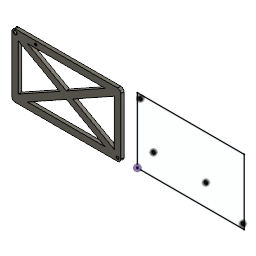
psu_mount_on_baseplate v1 (Autodesk Fusion 360 design; units mm, degrees)
Autodesk Fusion 360 part; units mm, degrees
sketch "Sketch1" plane through (0, 0, 0) normal (0, 0, 1) x (1, 0, 0)
  line L0 (100, 125) -> (-100, 125)
  line L1 (-100, 125) -> (-100, -125)
  line L2 (-100, -125) -> (100, -125)
  line L3 (100, -125) -> (100, 125)
  line L4 (100, 125) -> (-100, -125) construction
  line L5 (-100, 125) -> (100, -125) construction
  line L6 (-100, 125) -> (100, 125)
  line L7 (100, 125) -> (100, 129)
  line L8 (100, 129) -> (-100, 129)
  line L9 (-100, 129) -> (-100, 125)
  line L10 (-100, -125) -> (100, -125)
  line L11 (100, -125) -> (100, -129)
  line L12 (100, -129) -> (-100, -129)
  line L13 (-100, -129) -> (-100, -125)
  line L14 (100, 125) -> (104, 125)
  line L15 (104, 125) -> (104, -125)
  line L16 (104, -125) -> (100, -125)
  line L17 (100, -125) -> (100, 125)
  line L18 (-100, 125) -> (-104, 125)
  line L19 (-104, 125) -> (-104, -125)
  line L20 (-104, -125) -> (-100, -125)
  line L21 (-100, -125) -> (-100, 125)
  line L22 (-80, -53.8) -> (-80, 2.2) construction
  circle A0 centre (-80, -53.8) radius 1.65 construction
  circle A1 centre (-80, 2.2) radius 1.65 construction
  line L23 (-61.0622, -1) -> (-98.9378, -1) construction
  line L24 (-98.9378, -1) -> (-98.9378, -50.6) construction
  line L25 (-98.9378, -50.6) -> (-61.0622, -50.6) construction
  line L26 (-61.0622, -50.6) -> (-61.0622, -1) construction
  line L27 (-61.0622, -1) -> (-98.9378, -50.6) construction
  line L28 (-98.9378, -1) -> (-61.0622, -50.6) construction
  line L29 (-30.5, 49.5) -> (98.5, 49.5) construction
  line L30 (98.5, 49.5) -> (98.5, -47.5) construction
  line L31 (98.5, -47.5) -> (-30.5, -47.5) construction
  line L32 (-30.5, -47.5) -> (-30.5, 49.5) construction
  circle A2 centre (-28, 43) radius 1.65
  circle A3 centre (94, -42) radius 1.65
  line L33 (-100, 125) -> (-85.5, 125)
  line L34 (-85.5, 125) -> (-85.5, 116)
  line L35 (-85.5, 116) -> (-100, 116)
  line L36 (-100, 116) -> (-100, 125)
  line L37 (100, 125) -> (85.5, 125)
  line L38 (85.5, 125) -> (85.5, 116)
  line L39 (85.5, 116) -> (100, 116)
  line L40 (100, 116) -> (100, 125)
  line L41 (-100, -125) -> (-85.5, -125)
  line L42 (-85.5, -125) -> (-85.5, -116)
  line L43 (-85.5, -116) -> (-100, -116)
  line L44 (-100, -116) -> (-100, -125)
  line L45 (100, -125) -> (85.5, -125)
  line L46 (85.5, -125) -> (85.5, -116)
  line L47 (85.5, -116) -> (100, -116)
  line L48 (100, -116) -> (100, -125)
  line L49 (-100, 100) -> (-104, 100)
  line L50 (100, 100) -> (104, 100)
  line L51 (-100, -100) -> (-104, -100)
  line L52 (100, -100) -> (104, -100)
  line L53 (-85.5, 125) -> (-85.5, 129)
  line L54 (85.5, 125) -> (85.5, 129)
  line L55 (-85.5, -125) -> (-85.5, -129)
  line L56 (85.5, -125) -> (85.5, -129)
  line L57 (-115, -140) -> (-75, -140) construction
  line L58 (-75, -140) -> (-75, -87) construction
  line L59 (-75, -87) -> (-115, -87) construction
  line L60 (-115, -87) -> (-115, -140) construction
  line L61 (-63.3606, -140) -> (-21.3606, -140) construction
  line L62 (-21.3606, -140) -> (-21.3606, -53.8) construction
  line L63 (-21.3606, -53.8) -> (-63.3606, -53.8) construction
  line L64 (-63.3606, -53.8) -> (-63.3606, -140) construction
  line L65 (-100, 0) -> (-118.2487, 0) construction
  circle A4 centre (0, 0) radius 152.5
  circle A5 centre (-85, -72) radius 1.65
  line L66 (-85, -72) -> (85, -72) construction
  line L67 (85, -72) -> (85, 72) construction
  line L68 (85, 72) -> (-85, 72) construction
  line L69 (-85, 72) -> (-85, -72) construction
  circle A6 centre (85, 72) radius 1.65
  circle A7 centre (85, -72) radius 1.65
  circle A8 centre (-85, 72) radius 1.65
  point P0 (-80, -25.8)
  dimension "d1" = 200
  dimension "d2" = 250
  dimension "d3" = 4
  dimension "d4" = 4
  dimension "d5" = 4
  dimension "d6" = 4
  dimension "d7" = 20
  dimension "d8" = 56
  dimension "d10" = 3.3
  dimension "d11" = 37.8755
  dimension "d12" = 49.6
  dimension "d13" = 2.5
  dimension "d14" = 6.5
  dimension "d15" = 3.3
  dimension "d16" = 5.5
  dimension "d17" = 4.5
  dimension "d18" = 129
  dimension "d19" = 97
  dimension "d20" = 1.5
  dimension "d21" = 14.5
  dimension "d22" = 9
  dimension "d23" = 14.5
  dimension "d24" = 9
  dimension "d25" = 14.5
  dimension "d26" = 14.5
  dimension "d27" = 9
  dimension "d28" = 9
  dimension "d29" = 25
  dimension "d30" = 25
  dimension "d31" = 25
  dimension "d32" = 25
  dimension "d33" = 40
  dimension "d34" = 53
  dimension "d35" = 15
  dimension "d36" = 15
  dimension "d37" = 3.3
  dimension "d38" = 86.2
  dimension "d39" = 42
  dimension "d40" = 1
  dimension "d50" = 305
  dimension "d51" = 3.3
  dimension "d52" = 15
  dimension "d53" = 15
  dimension "d54" = 15
  dimension "d55" = 53
  dimension "d56" = 53
  dimension "d57" = 170
  dimension "d58" = 144
  dimension "d60" = 47.5
  dimension "d61" = 49.5
  constraint horizontal L0
  constraint perpendicular L0 L1
  constraint parallel L0 L2
  constraint parallel L1 L3
  constraint coincident L4 A4.centre
  constraint coincident L5 A4.centre
  constraint coincident A4.centre origin
  constraint horizontal L6
  constraint vertical L7
  constraint horizontal L8
  constraint vertical L9
  constraint horizontal L10
  constraint vertical L11
  constraint horizontal L12
  constraint vertical L13
  constraint horizontal L14
  constraint vertical L15
  constraint horizontal L16
  constraint vertical L17
  constraint horizontal L18
  constraint vertical L19
  constraint horizontal L20
  constraint vertical L21
  constraint coincident L22.start A0.centre
  constraint coincident L22.end A1.centre
  constraint equal A0 A1
  constraint horizontal L23
  constraint perpendicular L23 L24
  constraint parallel L23 L25
  constraint parallel L24 L26
  constraint coincident L27 P0
  constraint coincident L28 P0
  constraint midpoint L22 P0
  constraint collinear L2 L20
  constraint collinear L11 L17
  constraint collinear L7 L17
  constraint horizontal L29
  constraint vertical L30
  constraint horizontal L31
  constraint vertical L32
  constraint equal A2 A3
  constraint horizontal L33
  constraint vertical L34
  constraint horizontal L35
  constraint vertical L36
  constraint horizontal L37
  constraint vertical L38
  constraint horizontal L39
  constraint vertical L40
  constraint horizontal L41
  constraint vertical L42
  constraint horizontal L43
  constraint vertical L44
  constraint horizontal L45
  constraint vertical L46
  constraint horizontal L47
  constraint vertical L48
  constraint coincident L1 L49.start
  constraint coincident L19 L49.end
  constraint perpendicular L19 L49
  constraint coincident L3 L50.start
  constraint coincident L15 L50.end
  constraint perpendicular L15 L50
  constraint coincident L21 L51.start
  constraint coincident L19 L51.end
  constraint perpendicular L19 L51
  constraint coincident L17 L52.start
  constraint coincident L15 L52.end
  constraint perpendicular L15 L52
  constraint coincident L8 L53.end
  constraint perpendicular L8 L53
  constraint coincident L8 L54.end
  constraint perpendicular L8 L54
  constraint coincident L12 L55.end
  constraint perpendicular L12 L55
  constraint coincident L12 L56.end
  constraint perpendicular L12 L56
  constraint horizontal L57
  constraint vertical L58
  constraint horizontal L59
  constraint vertical L60
  constraint horizontal L61
  constraint vertical L62
  constraint horizontal L63
  constraint vertical L64
  constraint vertical L22
  constraint midpoint L21 L65.start
  constraint perpendicular L19 L65
  constraint collinear L57 L61
  constraint horizontal L66
  constraint vertical L67
  constraint horizontal L68
  constraint vertical L69
  constraint coincident A5.centre L66.start
  constraint coincident L67.end L68.start
  constraint coincident L66.end L67.start
  constraint coincident L68.end L69.start
  constraint equal A6 A8
  constraint equal A5 A7
  constraint equal A6 A7
  measures "d1" distance of L0.start L0.end
  measures "d2" distance of L0.start L2.end
  measures "d3" distance of L0 L8
  measures "d4" distance of L2.end L11.end
  measures "d5" distance of L0.start L14.end
  measures "d6" distance of L0.end L18.end
  measures "d7" distance of L1 L22.start
  measures "d8" distance of L22.start L22.end
  measures "d10" diameter of A1
  measures "d11" distance of L23.start L23.end
  measures "d12" distance of L23.start L25.end
  measures "d13" distance of L32 A2.centre
  measures "d14" distance of L29 A2.centre
  measures "d15" diameter of A2
  measures "d16" distance of L31 A3.centre
  measures "d17" distance of L30 A3.centre
  measures "d18" distance of L29.start L29.end
  measures "d19" distance of L29.end L30.end
  measures "d20" distance of L17 L30
  measures "d21" distance of L34.end L35.end
  measures "d22" distance of L33.end L34.end
  measures "d23" distance of L38.end L39.end
  measures "d24" distance of L37.end L38.end
  measures "d25" distance of L42.end L43.end
  measures "d26" distance of L46.end L47.end
  measures "d27" distance of L41.end L42.end
  measures "d28" distance of L45.end L46.end
  measures "d29" distance of L20 L51
  measures "d30" distance of L18 L49
  measures "d31" distance of L14 L50
  measures "d32" distance of L10 L52
  measures "d33" distance of L57.start L57.end
  measures "d34" distance of L57.start L59.end
  measures "d35" distance of L10 L57
  measures "d36" distance of L21 L60
  measures "d37" diameter of A3
  measures "d38" distance of L61.end L62.end
  measures "d39" distance of L61.start L61.end
  measures "d40" distance of L23 L65
  measures "d50" diameter of A4
  measures "d51" diameter of A5
  measures "d52" distance of L1 A5.centre
  measures "d53" distance of L59 A5.centre
  measures "d54" distance of L17 L67
  measures "d55" distance of L10 L66
  measures "d56" distance of L6 L68
  measures "d57" distance of L67.end L68.end
  measures "d58" distance of L66.end L67.end
  measures "d60" distance of L31 L65
  measures "d61" distance of L29 L65
extrude "Extrude1" add sketch "Sketch1" along normal blind 3 contours L0 L1 L2 L3 L6 L10 L17 L21 L34 L35 L38 L39 L42 L43 L46 L47 A4 | L0 L6 L8 L53 L54 A4 | L3 L15 L17 L50 L52 | L1 L19 L21 L49 L51 | L2 L10 L12 L55 L56 A4 makes body 1
sketch "Sketch2" plane through (0, 0, 3) normal (0, 0, 1) x (1, 0, 0)
  circle A0 centre (85, -72) radius 1.65
  circle A1 centre (-85, -72) radius 1.65
  circle A2 centre (85, 72) radius 1.65
  circle A3 centre (94, -42) radius 1.65
  circle A4 centre (-85, 72) radius 1.65
  circle A5 centre (-28, 43) radius 1.65
  line L0 (100, 100) -> (100, 115.1358)
  arc A6 (100, 115.1358) -> (98.9962, 116) centre (0, 0) ccw
  line L1 (98.9962, 116) -> (85.5, 116)
  line L2 (85.5, 116) -> (85.5, 126.2775)
  arc A7 (85.5, 126.2775) -> (81.3342, 129) centre (0, 0) ccw
  line L3 (81.3342, 129) -> (-81.3342, 129)
  arc A8 (-81.3342, 129) -> (-85.5, 126.2775) centre (0, 0) ccw
  line L4 (-85.5, 126.2775) -> (-85.5, 116)
  line L5 (-85.5, 116) -> (-98.9962, 116)
  arc A9 (-98.9962, 116) -> (-100, 115.1358) centre (0, 0) ccw
  line L6 (-100, 115.1358) -> (-100, 100)
  line L7 (-100, 100) -> (-104, 100)
  line L8 (-104, 100) -> (-104, -100)
  line L9 (-104, -100) -> (-100, -100)
  line L10 (-100, -100) -> (-100, -115.1358)
  arc A10 (-100, -115.1358) -> (-98.9962, -116) centre (0, 0) ccw
  line L11 (-98.9962, -116) -> (-85.5, -116)
  line L12 (-85.5, -116) -> (-85.5, -126.2775)
  arc A11 (-85.5, -126.2775) -> (-81.3342, -129) centre (0, 0) ccw
  line L13 (-81.3342, -129) -> (81.3342, -129)
  arc A12 (81.3342, -129) -> (85.5, -126.2775) centre (0, 0) ccw
  line L14 (85.5, -126.2775) -> (85.5, -116)
  line L15 (85.5, -116) -> (98.9962, -116)
  arc A13 (98.9962, -116) -> (100, -115.1358) centre (0, 0) ccw
  line L16 (100, -115.1358) -> (100, -100)
  line L17 (100, -100) -> (104, -100)
  line L18 (104, -100) -> (104, 100)
  line L19 (104, 100) -> (100, 100)
  line L20 (-10, 129) -> (10, 129)
  line L21 (10, 129) -> (10, 111)
  line L22 (8, 109) -> (-8, 109)
  line L23 (-10, 111) -> (-10, 129)
  arc A14 (-10, 111) -> (-8, 109) centre (-8, 111) ccw
  arc A15 (8, 109) -> (10, 111) centre (8, 111) ccw
  point P0 (10, 109)
  point P1 (-10, 109)
  dimension "d62" = 20
  dimension "d63" = 20
  dimension "d64" = 2
  constraint horizontal L20
  constraint vertical L21
  constraint horizontal L22
  constraint vertical L23
  constraint coincident L3 L20.start
  constraint midpoint L3 L20
  constraint coincident P1 L22
  constraint coincident P1 L23
  constraint tangent L22 A14
  constraint tangent L23 A14
  constraint coincident P0 L21
  constraint coincident P0 L22
  constraint tangent L21 A15
  constraint tangent L22 A15
  constraint equal A14 A15
  measures "d62" distance of L20.start P1
  measures "d63" distance of P0 P1
  measures "d64" radius of A14
extrude "Extrude2" cut sketch "Sketch2" against normal blind 3 contours L3 L20 L21 L22 L23 A14 A15 bodies 1
fillet "Fillet4" radius 2 2 edges at (-10, 129, 1.5) (10, 129, 1.5) on bodies 1
sketch "Sketch3" plane through (0, 0, 3) normal (0, 0, 1) x (1, 0, 0)
  arc A0 (12, 129) -> (10, 127) centre (12, 127) ccw
  line L0 (10, 127) -> (10, 111)
  arc A1 (8, 109) -> (10, 111) centre (8, 111) ccw
  line L1 (8, 109) -> (-8, 109)
  arc A2 (-10, 111) -> (-8, 109) centre (-8, 111) ccw
  line L2 (-10, 111) -> (-10, 127)
  arc A3 (-10, 127) -> (-12, 129) centre (-12, 127) ccw
  line L3 (-12, 129) -> (-81.3342, 129)
  arc A4 (-81.3342, 129) -> (-85.5, 126.2775) centre (0, 0) ccw
  line L4 (-85.5, 126.2775) -> (-85.5, 116)
  line L5 (-85.5, 116) -> (-98.9962, 116)
  arc A5 (-98.9962, 116) -> (-100, 115.1358) centre (0, 0) ccw
  line L6 (-100, 115.1358) -> (-100, 100)
  line L7 (-100, 100) -> (-104, 100)
  line L8 (-104, 100) -> (-104, -100)
  line L9 (-104, -100) -> (-100, -100)
  line L10 (-100, -100) -> (-100, -115.1358)
  arc A6 (-100, -115.1358) -> (-98.9962, -116) centre (0, 0) ccw
  line L11 (-98.9962, -116) -> (-85.5, -116)
  line L12 (-85.5, -116) -> (-85.5, -126.2775)
  arc A7 (-85.5, -126.2775) -> (-81.3342, -129) centre (0, 0) ccw
  line L13 (-81.3342, -129) -> (81.3342, -129)
  arc A8 (81.3342, -129) -> (85.5, -126.2775) centre (0, 0) ccw
  line L14 (85.5, -126.2775) -> (85.5, -116)
  line L15 (85.5, -116) -> (98.9962, -116)
  arc A9 (98.9962, -116) -> (100, -115.1358) centre (0, 0) ccw
  line L16 (100, -115.1358) -> (100, -100)
  line L17 (100, -100) -> (104, -100)
  line L18 (104, -100) -> (104, 100)
  line L19 (104, 100) -> (100, 100)
  line L20 (100, 100) -> (100, 115.1358)
  arc A10 (100, 115.1358) -> (98.9962, 116) centre (0, 0) ccw
  line L21 (98.9962, 116) -> (85.5, 116)
  line L22 (85.5, 116) -> (85.5, 126.2775)
  arc A11 (85.5, 126.2775) -> (81.3342, 129) centre (0, 0) ccw
  line L23 (81.3342, 129) -> (12, 129)
  circle A12 centre (85, -72) radius 1.65
  circle A13 centre (-85, -72) radius 1.65
  circle A14 centre (85, 72) radius 1.65
  circle A15 centre (94, -42) radius 1.65
  circle A16 centre (-85, 72) radius 1.65
  circle A17 centre (-28, 43) radius 1.65
  circle A18 centre (0, 59) radius 6
  dimension "d69" = 12
  dimension "d70" = 50
  dimension "d71" = 104
  measures "d69" diameter of A18
  measures "d70" distance of L1 A18.centre
  measures "d71" distance of L8 A18.centre
extrude "Extrude3" cut sketch "Sketch3" against normal blind 3 contours A18 bodies 1
sketch "Sketch4" plane through (0, 0, 3) normal (0, 0, 1) x (1, 0, 0)
  circle A0 centre (0, 59) radius 6
  arc A1 (12, 129) -> (10, 127) centre (12, 127) ccw
  line L0 (10, 127) -> (10, 111)
  arc A2 (8, 109) -> (10, 111) centre (8, 111) ccw
  line L1 (8, 109) -> (-8, 109)
  arc A3 (-10, 111) -> (-8, 109) centre (-8, 111) ccw
  line L2 (-10, 111) -> (-10, 127)
  arc A4 (-10, 127) -> (-12, 129) centre (-12, 127) ccw
  line L3 (-12, 129) -> (-81.3342, 129)
  arc A5 (-81.3342, 129) -> (-85.5, 126.2775) centre (0, 0) ccw
  line L4 (-85.5, 126.2775) -> (-85.5, 116)
  line L5 (-85.5, 116) -> (-98.9962, 116)
  arc A6 (-98.9962, 116) -> (-100, 115.1358) centre (0, 0) ccw
  line L6 (-100, 115.1358) -> (-100, 100)
  line L7 (-100, 100) -> (-104, 100)
  line L8 (-104, 100) -> (-104, -100)
  line L9 (-104, -100) -> (-100, -100)
  line L10 (-100, -100) -> (-100, -115.1358)
  arc A7 (-100, -115.1358) -> (-98.9962, -116) centre (0, 0) ccw
  line L11 (-98.9962, -116) -> (-85.5, -116)
  line L12 (-85.5, -116) -> (-85.5, -126.2775)
  arc A8 (-85.5, -126.2775) -> (-81.3342, -129) centre (0, 0) ccw
  line L13 (-81.3342, -129) -> (81.3342, -129)
  arc A9 (81.3342, -129) -> (85.5, -126.2775) centre (0, 0) ccw
  line L14 (85.5, -126.2775) -> (85.5, -116)
  line L15 (85.5, -116) -> (98.9962, -116)
  arc A10 (98.9962, -116) -> (100, -115.1358) centre (0, 0) ccw
  line L16 (100, -115.1358) -> (100, -100)
  line L17 (100, -100) -> (104, -100)
  line L18 (104, -100) -> (104, 100)
  line L19 (104, 100) -> (100, 100)
  line L20 (100, 100) -> (100, 115.1358)
  arc A11 (100, 115.1358) -> (98.9962, 116) centre (0, 0) ccw
  line L21 (98.9962, 116) -> (85.5, 116)
  line L22 (85.5, 116) -> (85.5, 126.2775)
  arc A12 (85.5, 126.2775) -> (81.3342, 129) centre (0, 0) ccw
  line L23 (81.3342, 129) -> (12, 129)
  circle A13 centre (85, -72) radius 1.65
  circle A14 centre (-85, -72) radius 1.65
  circle A15 centre (85, 72) radius 1.65
  circle A16 centre (94, -42) radius 1.65
  circle A17 centre (-85, 72) radius 1.65
  circle A18 centre (-28, 43) radius 1.65
sketch "Sketch1 (2)" plane through (0, 0, 0) normal (0, 0, 1) x (1, 0, 0) in component "LRS-150-24 PSU v1"
  line L0 (0, 0) -> (159, 0)
  line L1 (159, 0) -> (159, 97)
  line L2 (159, 97) -> (0, 97)
  line L3 (0, 97) -> (0, 0)
  circle A0 centre (4.5, 91.5) radius 1.75
  circle A1 centre (24, 32) radius 1.75
  circle A2 centre (102, 32) radius 1.75
  circle A3 centre (157, 6.5) radius 1.75
  dimension "d1_1" = 159
  dimension "d2_1" = 97
  dimension "d3_1" = 3.5
  dimension "d4_1" = 3.5
  dimension "d5_1" = 3.5
  dimension "d6_1" = 3.5
  dimension "d7_1" = 4.5
  dimension "d8_1" = 91.5
  dimension "d9" = 24
  dimension "d10_1" = 32
  dimension "d11_1" = 102
  dimension "d12_1" = 32
  dimension "d13_1" = 6.5
  dimension "d14_1" = 157
  dimension "d14_1" = 157
  constraint horizontal L0
  constraint vertical L1
  constraint horizontal L2
  constraint vertical L3
  constraint coincident L0.start L3.end
  measures "d1_1" distance of L0.start L0.end
  measures "d2_1" distance of L0.start L2.end
  measures "d3_1" diameter of A0
  measures "d4_1" diameter of A1
  measures "d5_1" diameter of A2
  measures "d6_1" diameter of A3
  measures "d7_1" distance of L3 A0.centre
  measures "d8_1" distance of L0 A0.centre
  measures "d9" distance of L3 A1.centre
  measures "d10_1" distance of L0 A1.centre
  measures "d11_1" distance of L3 A2.centre
  measures "d12_1" distance of L0 A2.centre
  measures "d13_1" distance of L0 A3.centre
  measures "d14_1" distance of L3 A3.centre
sketch "Sketch6" plane through (0, 0, 3) normal (0, 0, 1) x (1, 0, 0)
  circle A0 centre (0, 59) radius 6
  arc A1 (12, 129) -> (10, 127) centre (12, 127) ccw
  line L0 (10, 127) -> (10, 111)
  arc A2 (8, 109) -> (10, 111) centre (8, 111) ccw
  line L1 (8, 109) -> (-8, 109)
  arc A3 (-10, 111) -> (-8, 109) centre (-8, 111) ccw
  line L2 (-10, 111) -> (-10, 127)
  arc A4 (-10, 127) -> (-12, 129) centre (-12, 127) ccw
  line L3 (-12, 129) -> (-81.3342, 129)
  arc A5 (-81.3342, 129) -> (-85.5, 126.2775) centre (0, 0) ccw
  line L4 (-85.5, 126.2775) -> (-85.5, 116)
  line L5 (-85.5, 116) -> (-98.9962, 116)
  arc A6 (-98.9962, 116) -> (-100, 115.1358) centre (0, 0) ccw
  line L6 (-100, 115.1358) -> (-100, 100)
  line L7 (-100, 100) -> (-104, 100)
  line L8 (-104, 100) -> (-104, -100)
  line L9 (-104, -100) -> (-100, -100)
  line L10 (-100, -100) -> (-100, -115.1358)
  arc A7 (-100, -115.1358) -> (-98.9962, -116) centre (0, 0) ccw
  line L11 (-98.9962, -116) -> (-85.5, -116)
  line L12 (-85.5, -116) -> (-85.5, -126.2775)
  arc A8 (-85.5, -126.2775) -> (-81.3342, -129) centre (0, 0) ccw
  line L13 (-81.3342, -129) -> (81.3342, -129)
  arc A9 (81.3342, -129) -> (85.5, -126.2775) centre (0, 0) ccw
  line L14 (85.5, -126.2775) -> (85.5, -116)
  line L15 (85.5, -116) -> (98.9962, -116)
  arc A10 (98.9962, -116) -> (100, -115.1358) centre (0, 0) ccw
  line L16 (100, -115.1358) -> (100, -100)
  line L17 (100, -100) -> (104, -100)
  line L18 (104, -100) -> (104, 100)
  line L19 (104, 100) -> (100, 100)
  line L20 (100, 100) -> (100, 115.1358)
  arc A11 (100, 115.1358) -> (98.9962, 116) centre (0, 0) ccw
  line L21 (98.9962, 116) -> (85.5, 116)
  line L22 (85.5, 116) -> (85.5, 126.2775)
  arc A12 (85.5, 126.2775) -> (81.3342, 129) centre (0, 0) ccw
  line L23 (81.3342, 129) -> (12, 129)
  circle A13 centre (85, -72) radius 1.65
  circle A14 centre (-85, -72) radius 1.65
  circle A15 centre (85, 72) radius 1.65
  circle A16 centre (94, -42) radius 1.65
  circle A17 centre (-85, 72) radius 1.65
  circle A18 centre (-28, 43) radius 1.65
  line L24 (94, -42) -> (-105.8448, -42) construction
  line L25 (94, -42) -> (104, -42) construction
  line L26 (-28, 43) -> (-104, 43) construction
  line L27 (-28, 43) -> (104, 43) construction
  line L28 (-28, 43) -> (-28, -42) construction
  line L29 (94, -42) -> (94, 43) construction
  circle A19 centre (-58.5, 43) radius 1.65
  circle A20 centre (-58.5, 43) radius 2.35
  circle A21 centre (-58.5, 43) radius 4.85
  circle A22 centre (94, -42) radius 4.85
  line L30 (89.15, -42) -> (89.15, 43)
  line L31 (-63.35, 43) -> (-63.35, -42)
  line L32 (-53.65, 43) -> (-53.65, -42)
  line L33 (94, -46.85) -> (-62.05, -46.85)
  line L34 (-63.35, -45.55) -> (-63.35, -42)
  line L35 (-53.65, -42) -> (-53.65, -46.85)
  line L36 (94, -37.15) -> (-63.35, -37.15)
  line L37 (-58.5, 38.15) -> (89.15, 38.15)
  line L38 (-58.5, 47.85) -> (98.85, 47.85)
  line L39 (89.15, 43) -> (89.15, 47.85)
  line L40 (89.15, 38.15) -> (98.85, 38.15)
  arc A23 (-63.35, -45.55) -> (-62.05, -46.85) centre (-62.05, -45.55) ccw
  line L41 (-60.8613, 38.7636) -> (91.6387, -46.2364)
  line L42 (96.3613, -37.7636) -> (-56.1387, 47.2364)
  circle A24 centre (-58.5709, -42) radius 4.85
  circle A25 centre (94, 43) radius 4.85
  line L43 (96.3604, 38.7632) -> (-56.2104, -46.2368)
  line L44 (-60.9313, -37.7632) -> (91.0575, 46.9126)
  line L45 (98.85, -42) -> (98.85, 43)
  line L46 (98.8483, 43.1271) -> (98.85, 47.85)
  circle A26 centre (-28, 43) radius 1.65
  circle A27 centre (-28, 43) radius 2.35
  circle A28 centre (-28, 43) radius 4.85
  dimension "d77" = 3.3
  dimension "d78" = 152.5
  dimension "d79" = 4.7
  dimension "d80" = 9.7
  dimension "d81" = 9.7
  dimension "d82" = 1.3
  dimension "d83" = 9.7
  dimension "d84" = 9.7
  dimension "d87" = 3.3
  dimension "d88" = 4.7
  dimension "d89" = 9.7
  constraint coincident A16.centre L24.start
  constraint perpendicular L8 L24
  constraint coincident L18 L25.end
  constraint perpendicular L18 L25
  constraint coincident A18.centre L26.start
  constraint coincident L8 L26.end
  constraint perpendicular L8 L26
  constraint coincident L18 L27.end
  constraint perpendicular L18 L27
  constraint coincident L24 L28.end
  constraint perpendicular L24 L28
  constraint coincident L27 L29.end
  constraint perpendicular L27 L29
  constraint coincident L26 A19.centre
  constraint concentric A19 A20
  constraint concentric A20 A21
  constraint coincident A22 L30.start
  constraint coincident L24 L30.start
  constraint coincident L27 L30.end
  constraint tangent A22 L30
  constraint coincident A21 L31.start
  constraint coincident L26 L31.start
  constraint coincident L24 L31.end
  constraint tangent A21 L31
  constraint coincident A21 L32.start
  constraint coincident L26 L32.start
  constraint coincident L24 L32.end
  constraint tangent A21 L32
  constraint coincident A22 L33.start
  constraint perpendicular L28 L33
  constraint perpendicular L24 L34
  constraint coincident L33 L35.end
  constraint perpendicular L33 L35
  constraint coincident A22 L36.start
  constraint coincident L29 L36.start
  constraint coincident L31 L36.end
  constraint tangent A22 L36
  constraint coincident A21 L37.start
  constraint coincident L30 L37.end
  constraint perpendicular L30 L37
  constraint coincident A21 L38.start
  constraint perpendicular L18 L38
  constraint coincident L38 L39.end
  constraint perpendicular L38 L39
  constraint tangent A21 L37
  constraint tangent A21 L38
  constraint tangent A22 L33
  constraint tangent L33 A23
  constraint tangent L34 A23
  constraint coincident A21 L41.start
  constraint coincident A22 L41.end
  constraint coincident A22 L42.start
  constraint coincident A21 L42.end
  constraint tangent A21 L42
  constraint tangent A21 L41
  constraint tangent A22 L41
  constraint tangent A22 L42
  constraint coincident L24 A24.centre
  constraint coincident L29.end A25.centre
  constraint coincident A25 L43.start
  constraint coincident A24 L43.end
  constraint coincident A24 L44.start
  constraint tangent A24 L44
  constraint tangent A25 L44
  constraint tangent A25 L43
  constraint tangent A24 L43
  constraint horizontal L40
  constraint coincident A22 L45.start
  constraint coincident L25 L45.start
  constraint tangent A22 L45
  constraint coincident A25 L46.start
  constraint coincident L40.end L45
  constraint concentric A26 A27
  constraint concentric A26 A28
  measures "d77" diameter of A19
  measures "d78" horizontal distance of A16.centre A19.centre
  measures "d79" diameter of A20
  measures "d80" diameter of A21
  measures "d81" diameter of A22
  measures "d82" radius of A23
  measures "d83" diameter of A24
  measures "d84" diameter of A25
  measures "d87" diameter of A26
  measures "d88" diameter of A27
  measures "d89" diameter of A28
extrude "Extrude4" add sketch "Sketch6" along normal blind 5 separate body contours A21 | A21 L32 L37 | A21 L32 L37 L42 | A21 L37 L38 L42 A28 | A21 L32 L37 L41 | L32 L37 L41 L42 L44 | A21 L31 L32 L36 L41 L44 | L37 L38 L39 L44 A28 | A28 | L30 L37 L42 L43 L44 | L41 L42 L43 L44 | L32 L36 L41 L43 L44 | L32 L36 L44 | L31 L36 A24 L44 | L38 L39 A25 | L30 L37 L39 L44 | L30 L36 L41 L42 L43 | L32 L35 L36 L43 | L32 L35 L36 A24 L43 | L36 A24 L44 | L31 L34 A24 | A25 | L30 L40 L43 | L30 L40 A25 | A22 L30 L36 L42 | A22 L30 L40 L42 L43 L45 | A22 L33 L35 L36 L41 L43 | A22 L30 L36 L41 | L40 A25 L43 | A22 L30 L36 | A22 | L40 A25 L43 L45 | L33 L35 A24 L43 | A27 picked at (-56.947, -41.7699) makes body 2
extrude "Extrude5" add sketch "Sketch6" along normal blind 1 contours A20 bodies 2
extrude "Extrude6" cut sketch "Sketch6" along normal blind 4 contours A27 bodies 1 2
fillet "Fillet5" radius 0.4 4 edges at (-60.691, 43.8498, 8) (92.4617, -41.4033, 8) (92.4617, -41.4033, 3) (-30.191, 42.1502, 3) on bodies 2
component "LRS-150-24 PSU v1" placed x (1, 0, 0) y (0, 1, 0) z (0, 0, 1) at (115.4323, -48.3981, 0)
hidden bodies 1
equation "d4 = d3"
equation "d5 = d3"
equation "d6 = d3"
equation "d23 = d21"
equation "d24 = d22"
equation "d25 = d21"
equation "d26 = d25"
equation "d27 = d22"
equation "d28 = d24"
equation "d30 = d29"
equation "d31 = d29"
equation "d32 = d29"
equation "d36 = d35"
equation "d60 = d19 / 2 - 1 mm"
equation "inner_heat = 3.3 mm"
equation "outer_heat = 4.7 mm"
equation "offset = 5 mm"
equation "d77 = inner_heat"
equation "d79 = outer_heat"
equation "d80 = outer_heat + offset"
equation "d81 = outer_heat + offset"
equation "d83 = outer_heat + offset"
equation "d84 = outer_heat + offset"
equation "d87 = inner_heat"
equation "d88 = outer_heat"
equation "d89 = outer_heat + offset"
equation "d8_1 = 85 mm + 6.5 mm"
equation "d11_1 = 24 mm + 78 mm"
equation "d14_1 = 4.5 mm + 152.5 mm"
equation "d14_1 = 4.5 mm + 152.5 mm"
